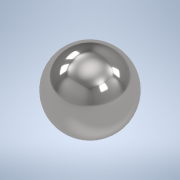
# Autodesk Inventor part: marble
Saved by Autodesk Inventor 2020 (Build 240168000, 168)
## iProperties
Created: 2021-03-06
Part Number: marble
Material: Generic
Document SubType Name: Modeling
Designer: Harry
Density: 1 g/cm^3
Appearance: Knurled 45
Author: Harry
Autodesk Inventor part; units mm, degrees
ref_plane "YZ Plane" through (0, 0, 0) normal (1, 0, 0) x (0, 1, 0)
ref_plane "XZ Plane" through (0, 0, 0) normal (0, 1, 0) x (-1, 0, 0)
ref_plane "XY Plane" through (0, 0, 0) normal (0, 0, 1) x (1, 0, 0)
sketch "Sketch1" plane through (0, 0, 0) normal (0, 0, 1) x (1, 0, 0)
  arc A0 (5, 0) -> (-5, 0) centre (0, 0) ccw
  line L0 (5, 0) -> (-5, 0)
  dimension "d0" = 10
  constraints: 2 end point, 2 point on circle, 1 centre point, 1 coincident, 1 horizontal
  measures "d0" diameter of A0
revolve "Revolution1" add sketch "Sketch1" angle 360 about axis through (5, 0, 0) along (-1, 0, 0)
body "Solid1"
